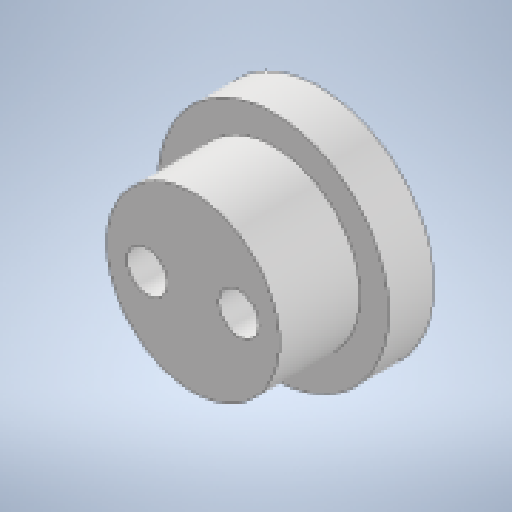
# Autodesk Inventor part: Shaft-4
Saved by Autodesk Inventor 2023 (Build 270158000, 158)
## iProperties
Created: 2023-01-17
Part Number: Shaft-4
Material: Generic
Document SubType Name: Modeling
Designer: caden
Density: 1 g/cm^3
Appearance: Default
Author: caden
Autodesk Inventor part; units mm, degrees
ref_plane "YZ Plane" through (0, 0, 0) normal (1, 0, 0) x (0, 1, 0)
ref_plane "XZ Plane" through (0, 0, 0) normal (0, 1, 0) x (-1, 0, 0)
ref_plane "XY Plane" through (0, 0, 0) normal (0, 0, 1) x (1, 0, 0)
sketch "Sketch1" plane through (0, 0, 0) normal (0, 0, 1) x (1, 0, 0)
  circle A0 centre (-5.747, 9.8039) radius 1.75
  circle A1 centre (-13.7036, 8.9717) radius 1.75
  line L0 (-5.747, 9.8039) -> (-13.7036, 8.9717) construction
  line L1 (-9.7253, 9.3878) -> (-8.5364, -1.9796) construction
  circle A2 centre (-9.7253, 9.3878) radius 10
  circle A3 centre (-9.4808, 7.9862) radius 7.5 projected
  circle A4 centre (-9.4808, 7.9862) radius 7.5 projected
  circle A5 centre (-13.4, 9.1649) radius 1.75 projected
  circle A6 centre (-13.4, 9.1649) radius 1.75 projected
  circle A7 centre (-5.8107, 9.7972) radius 1.75 projected
  circle A8 centre (-5.8107, 9.7972) radius 1.75 projected
  point P0 (0, 0)
  point P1 (-9.7132, 7.8251)
  dimension "d0" = 20
  dimension "d6" = 8
  constraints: 4 end point, 3 centre point, 2 midpoint, 1 perpendicular, 1 point on line
  measures "d0" diameter of A2
  measures "d6" distance of L0.start L0.end
extrude "Extrusion1" add sketch "Sketch1" along normal blind 3.9473 contours A0 A7 | A1 A5 | A2 | A3 picked at (-7.5243, 9.6868) picked at (-12.1064, 10.1413)
sketch "Sketch2" plane through (-9.7253, 9.3878, 3.9473) normal (0, 0, 1) x (1, 0, 0)
  circle A0 centre (0, 0) radius 7.5
  circle A1 centre (3.9783, 0.4161) radius 1.75 projected
  circle A2 centre (3.9783, 0.4161) radius 1.75
  circle A3 centre (-3.9783, -0.4161) radius 1.75 projected
  circle A4 centre (-3.9783, -0.4161) radius 1.75
  point P0 (9.7253, -9.3878)
  dimension "d3" = 15
  constraints: 3 centre point, 2 coincident
  measures "d3" diameter of A0
extrude "Extrusion2" add sketch "Sketch2" along normal blind 7
body "Solid1"
